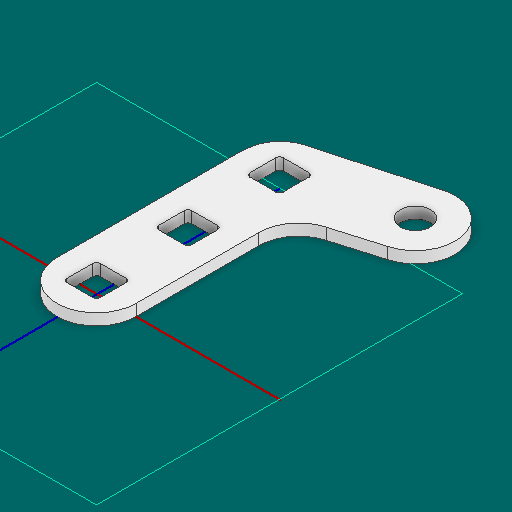
# Autodesk Inventor part: bent_gusset
Saved by Autodesk Inventor 2025 (Build 290162000, 162)
## iProperties
Created: 2024-08-16
Part Number: bent_gusset
Material: Acetal Resin, White
Document SubType Name: Modeling
Designer: averey
Density: 1.425 g/cm^3
Appearance: Smooth - White
Author: averey
Autodesk Inventor part; units mm, degrees
ref_plane "YZ Plane" through (0, 0, 0) normal (1, 0, 0) x (0, 1, 0)
ref_plane "XZ Plane" through (0, 0, 0) normal (0, 1, 0) x (-1, 0, 0)
ref_plane "XY Plane" through (0, 0, 0) normal (0, 0, 1) x (1, 0, 0)
sketch "main" plane through (0, 0, 0) normal (0, 0, 1) x (1, 0, 0)
  line L0 (-3.1973, -8.3156) -> (0.4095, -8.3156)
  arc A0 (-3.1973, -8.3156) -> (-3.7053, -8.8236) centre (-3.1973, -8.8236) ccw
  arc A1 (0.9175, -8.8236) -> (0.4095, -8.3156) centre (0.4095, -8.8236) ccw
  line L1 (-3.7053, -12.4304) -> (-3.7053, -8.8236)
  line L2 (0.9175, -8.8236) -> (0.9175, -12.4304)
  arc A2 (-3.7053, -12.4304) -> (-3.1973, -12.9384) centre (-3.1973, -12.4304) ccw
  line L3 (0.4095, -12.9384) -> (-3.1973, -12.9384)
  arc A3 (0.4095, -12.9384) -> (0.9175, -12.4304) centre (0.4095, -12.4304) ccw
  spline S0 degree 3 poles (4.1061, -10.627) (4.0635, -11.3826) (3.9418, -12.8881) (2.5369, -15.0176) (0.7715, -15.9468) (-0.3245, -16.1781) (-0.6942, -16.259) knots 0 0 0 0 0.294694 0.589389 0.884083 1.03143 1.03143 1.03143 1.03143
  arc A4 (-10.9164, -7.5728) -> (-6.8939, -2.275) centre (-12.3939, -2.275) ccw
  line L4 (-14.5376, -20.1198) -> (-0.6942, -16.259)
  line L5 (-10.9164, -7.5728) -> (-17.5138, -9.5303)
  arc A5 (-17.5138, -9.5303) -> (-14.5376, -20.1198) centre (-16.0578, -14.834) ccw
  circle A6 centre (-16.0578, -14.834) radius 2.1
  line L6 (0.4095, -0.2384) -> (-3.1973, -0.2384)
  arc A7 (-3.7053, 0.2696) -> (-3.1973, -0.2384) centre (-3.1973, 0.2696) ccw
  line L7 (0.9175, 3.8764) -> (0.9175, 0.2696)
  line L8 (-3.7053, 0.2696) -> (-3.7053, 3.8764)
  line L9 (-3.1973, 4.3844) -> (0.4095, 4.3844)
  arc A8 (-3.1973, 4.3844) -> (-3.7053, 3.8764) centre (-3.1973, 3.8764) ccw
  arc A9 (0.9175, 3.8764) -> (0.4095, 4.3844) centre (0.4095, 3.8764) ccw
  arc A10 (0.4095, -0.2384) -> (0.9175, 0.2696) centre (0.4095, 0.2696) ccw
  line L10 (4.1061, -10.627) -> (4.1061, 14.773)
  arc A11 (4.1061, 14.773) -> (-6.8939, 14.773) centre (-1.3939, 14.773) ccw
  line L11 (-6.8939, 14.773) -> (-6.8939, -2.275)
  line L12 (0.4095, 12.4616) -> (-3.1973, 12.4616)
  arc A12 (0.4095, 12.4616) -> (0.9175, 12.9696) centre (0.4095, 12.9696) ccw
  arc A13 (-3.7053, 12.9696) -> (-3.1973, 12.4616) centre (-3.1973, 12.9696) ccw
  line L13 (0.9175, 16.5764) -> (0.9175, 12.9696)
  line L14 (-3.7053, 12.9696) -> (-3.7053, 16.5764)
  arc A14 (-3.1973, 17.0844) -> (-3.7053, 16.5764) centre (-3.1973, 16.5764) ccw
  arc A15 (0.9175, 16.5764) -> (0.4095, 17.0844) centre (0.4095, 16.5764) ccw
  line L15 (-3.1973, 17.0844) -> (0.4095, 17.0844)
  line L16 (-15.2156, -14.4817) -> (-14.3027, -14.4817) construction
  point P0 (-2.9609, 0.4438)
  point P1 (-20.5005, 14.8552)
  dimension "d8" = 5.5
  measures "d8" radius of A5
sketch "Sketch1" plane through (0, 0, 0) normal (0, 1, 0) x (-1, 0, 0)
  line L0 (-1.8034, -23.0886) -> (1.8034, -23.0886)
  arc A0 (-1.8034, -23.0886) -> (-2.3114, -23.5966) centre (-1.8034, -23.5966) ccw
  arc A1 (2.3114, -23.5966) -> (1.8034, -23.0886) centre (1.8034, -23.5966) ccw
  line L1 (-2.3114, -27.2034) -> (-2.3114, -23.5966)
  line L2 (2.3114, -23.5966) -> (2.3114, -27.2034)
  arc A2 (-2.3114, -27.2034) -> (-1.8034, -27.7114) centre (-1.8034, -27.2034) ccw
  line L3 (1.8034, -27.7114) -> (-1.8034, -27.7114)
  arc A3 (1.8034, -27.7114) -> (2.3114, -27.2034) centre (1.8034, -27.2034) ccw
  spline S0 degree 3 poles (5.5, -25.4) (5.4573, -26.1557) (5.3357, -27.6611) (3.9308, -29.7907) (2.1654, -30.7198) (1.0693, -30.9511) (0.6997, -31.0321) knots 0 0 0 0 0.294694 0.589389 0.884083 1.03143 1.03143 1.03143 1.03143
  arc A4 (-9.5225, -22.3458) -> (-5.5, -17.048) centre (-11, -17.048) ccw
  line L4 (-13.1438, -34.8928) -> (0.6997, -31.0321)
  line L5 (-9.5225, -22.3458) -> (-16.12, -24.3033)
  arc A5 (-16.12, -24.3033) -> (-13.1438, -34.8928) centre (-14.6639, -29.6071) ccw
  circle A6 centre (-14.6639, -29.6071) radius 2.1
  line L6 (1.8034, -15.0114) -> (-1.8034, -15.0114)
  arc A7 (-2.3114, -14.5034) -> (-1.8034, -15.0114) centre (-1.8034, -14.5034) ccw
  line L7 (2.3114, -10.8966) -> (2.3114, -14.5034)
  line L8 (-2.3114, -14.5034) -> (-2.3114, -10.8966)
  line L9 (-1.8034, -10.3886) -> (1.8034, -10.3886)
  arc A8 (-1.8034, -10.3886) -> (-2.3114, -10.8966) centre (-1.8034, -10.8966) ccw
  arc A9 (2.3114, -10.8966) -> (1.8034, -10.3886) centre (1.8034, -10.8966) ccw
  arc A10 (1.8034, -15.0114) -> (2.3114, -14.5034) centre (1.8034, -14.5034) ccw
  line L10 (5.5, -25.4) -> (5.5, 0)
  arc A11 (5.5, 0) -> (-5.5, 0) centre (0, 0) ccw
  line L11 (-5.5, 0) -> (-5.5, -17.048)
  line L12 (1.8034, -2.3114) -> (-1.8034, -2.3114)
  arc A12 (1.8034, -2.3114) -> (2.3114, -1.8034) centre (1.8034, -1.8034) ccw
  arc A13 (-2.3114, -1.8034) -> (-1.8034, -2.3114) centre (-1.8034, -1.8034) ccw
  line L13 (2.3114, 1.8034) -> (2.3114, -1.8034)
  line L14 (-2.3114, -1.8034) -> (-2.3114, 1.8034)
  arc A14 (-1.8034, 2.3114) -> (-2.3114, 1.8034) centre (-1.8034, 1.8034) ccw
  arc A15 (2.3114, 1.8034) -> (1.8034, 2.3114) centre (1.8034, 1.8034) ccw
  line L15 (-1.8034, 2.3114) -> (1.8034, 2.3114)
  line L16 (-13.8217, -29.2547) -> (-12.9088, -29.2547) construction
  constraints: 1 other
extrude "Extrusion1" add sketch "Sketch1" along normal blind 1.5875
body "Solid1"
